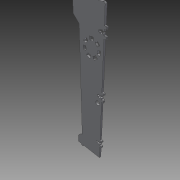
# Autodesk Inventor part: inner_brace_right
Saved by Autodesk Inventor 2014 (Build 180170000, 170)
## iProperties
Created: 2014-03-31
Part Number: inner_brace_right
Material: Plywood, Finish
Document SubType Name: Modeling
Designer: buben
Density: 0.552 g/cm^3
Appearance: Plywood - New
Author: buben
Autodesk Inventor part; units mm, degrees
ref_plane "YZ Plane" through (0, 0, 0) normal (1, 0, 0) x (0, 1, 0)
ref_plane "XZ Plane" through (0, 0, 0) normal (0, 1, 0) x (-1, 0, 0)
ref_plane "XY Plane" through (0, 0, 0) normal (0, 0, 1) x (1, 0, 0)
sketch "Sketch1" plane through (0, 0, 0) normal (0, 1, 0) x (-1, 0, 0)
  line L0 (0, 0) -> (-100, 0)
  line L1 (-100, 0) -> (-100, -489)
  line L2 (-100, -489) -> (0, -489)
  line L3 (0, -489) -> (0, 0)
  dimension "d0" = 489
  dimension "d1" = 100
  constraints: 8 end point, 2 parallel, 1 horizontal, 1 perpendicular
  measures "d0" distance of L2.end L0.start
  measures "d1" distance of L0.start L0.end
extrude "Extrusion1" add sketch "Sketch1" along normal blind 6.5
sketch "Sketch2" plane through (0, 6.5, 0) normal (0, 1, 0) x (1, 0, 0)
  line L0 (0, 489) -> (0, 0) projected
  line L1 (0, 459) -> (20, 439)
  line L2 (20, 439) -> (20, 65)
  line L3 (20, 65) -> (0, 45)
  line L4 (0, 459) -> (0, 45)
  dimension "d4" = 45
  dimension "d5" = 20
  dimension "d6" = 30
  dimension "d7" = 45
  constraints: 8 end point, 2 parallel, 2 point on line, 1 perpendicular
  measures "d4" angle of L0 L1
  measures "d5" distance between parallel lines of L0 L2
  measures "d6" distance of L0.start L1.start
  measures "d7" distance of L0.end L3.end
extrude "Extrusion2" cut sketch "Sketch2" against normal through all
sketch "Sketch3" plane through (0, 6.5, 0) normal (0, 1, 0) x (1, 0, 0)
  line L0 (0, 0) -> (100, 0) projected
  line L1 (100, 0) -> (100, 489) projected
  line L2 (100, 489) -> (0, 489) projected
  line L3 (100, 425.75) -> (100, 421.25)
  line L4 (83.7, 421.25) -> (83.7, 425.75)
  line L5 (87.7, 428.25) -> (95, 428.25)
  line L6 (95, 418.75) -> (87.7, 418.75)
  line L7 (83.7, 425.75) -> (87.7, 425.75)
  line L8 (95, 425.75) -> (100, 425.75)
  line L9 (87.7, 418.75) -> (87.7, 421.25)
  line L10 (87.7, 425.75) -> (87.7, 428.25)
  line L11 (100, 421.25) -> (95, 421.25)
  line L12 (87.7, 421.25) -> (83.7, 421.25)
  line L13 (95, 428.25) -> (95, 425.75)
  line L14 (95, 421.25) -> (95, 418.75)
  line L15 (100, 246.75) -> (100, 242.25)
  line L16 (83.7, 242.25) -> (83.7, 246.75)
  line L17 (87.7, 249.25) -> (95, 249.25)
  line L18 (95, 239.75) -> (87.7, 239.75)
  line L19 (83.7, 246.75) -> (87.7, 246.75)
  line L20 (95, 246.75) -> (100, 246.75)
  line L21 (87.7, 239.75) -> (87.7, 242.25)
  line L22 (87.7, 246.75) -> (87.7, 249.25)
  line L23 (100, 242.25) -> (95, 242.25)
  line L24 (87.7, 242.25) -> (83.7, 242.25)
  line L25 (95, 249.25) -> (95, 246.75)
  line L26 (95, 242.25) -> (95, 239.75)
  line L27 (100, 67.75) -> (100, 63.25)
  line L28 (83.7, 63.25) -> (83.7, 67.75)
  line L29 (87.7, 70.25) -> (95, 70.25)
  line L30 (95, 60.75) -> (87.7, 60.75)
  line L31 (83.7, 67.75) -> (87.7, 67.75)
  line L32 (95, 67.75) -> (100, 67.75)
  line L33 (87.7, 60.75) -> (87.7, 63.25)
  line L34 (87.7, 67.75) -> (87.7, 70.25)
  line L35 (100, 63.25) -> (95, 63.25)
  line L36 (87.7, 63.25) -> (83.7, 63.25)
  line L37 (95, 70.25) -> (95, 67.75)
  line L38 (95, 63.25) -> (95, 60.75)
  line L39 (91.35, 418.75) -> (91.35, 249.25) construction
  line L40 (91.35, 239.75) -> (91.35, 70.25) construction
  point P0 (83.7, 423.5)
  point P1 (83.7, 244.5)
  point P2 (83.7, 65.5)
  dimension "d10" = 4.5
  dimension "d11" = 5
  dimension "d12" = 4
  dimension "d13" = 7.3
  dimension "d14" = 2.5
  dimension "d15" = 4.5
  dimension "d16" = 5
  dimension "d17" = 4
  dimension "d18" = 7.3
  dimension "d19" = 2.5
  dimension "d20" = 4.5
  dimension "d21" = 5
  dimension "d22" = 4
  dimension "d23" = 7.3
  dimension "d24" = 2.5
  dimension "d25" = 65.5
  dimension "d26" = 65.5
  constraints: 76 end point, 30 parallel, 19 collinear, 12 perpendicular, 9 horizontal, 7 midpoint
  measures "d10" distance of L4.start L4.end
  measures "d11" distance of L3.end L11.end
  measures "d12" distance of L9.end L4.start
  measures "d13" distance of L6.start L6.end
  measures "d14" distance of L6.end L9.end
  measures "d15" distance of L24.end L16.end
  measures "d16" distance of L15.end L23.end
  measures "d17" distance of L21.end L24.end
  measures "d18" distance of L26.end L21.start
  measures "d19" distance of L21.start L21.end
  measures "d20" distance of L36.end L28.end
  measures "d21" distance of L27.end L35.end
  measures "d22" distance of L33.end L36.end
  measures "d23" distance of L38.end L33.start
  measures "d24" distance of L33.start L33.end
  measures "d25" distance from line of L2 point (83.7, 423.5)
  measures "d26" distance from line of L0 point (83.7, 65.5)
extrude "Extrusion3" cut sketch "Sketch3" against normal through all
sketch "Sketch4" plane through (0, 6.5, 0) normal (0, 1, 0) x (1, 0, 0)
  line L0 (83.7, 242.25) -> (83.7, 246.75) projected
  line L1 (100, 246.75) -> (100, 421.25) projected
  line L2 (83.7, 421.25) -> (83.7, 425.75) projected
  line L3 (100, 425.75) -> (100, 489) projected
  line L4 (100, 0) -> (100, 63.25) projected
  line L5 (83.7, 63.25) -> (83.7, 67.75) projected
  line L6 (100, 67.75) -> (100, 242.25) projected
  line L7 (100, 439) -> (104.5, 439)
  line L8 (106.5, 437) -> (106.5, 433)
  line L9 (104.5, 431) -> (100, 431)
  line L10 (100, 431) -> (100, 439)
  line L11 (100, 416) -> (104.5, 416)
  line L12 (106.5, 414) -> (106.5, 410)
  line L13 (104.5, 408) -> (100, 408)
  line L14 (100, 408) -> (100, 416)
  line L15 (100, 260) -> (104.5, 260)
  line L16 (106.5, 258) -> (106.5, 254)
  line L17 (104.5, 252) -> (100, 252)
  line L18 (100, 252) -> (100, 260)
  line L19 (100, 237) -> (104.5, 237)
  line L20 (106.5, 235) -> (106.5, 231)
  line L21 (104.5, 229) -> (100, 229)
  line L22 (100, 229) -> (100, 237)
  line L23 (100, 81) -> (104.5, 81)
  line L24 (106.5, 79) -> (106.5, 75)
  line L25 (104.5, 73) -> (100, 73)
  line L26 (100, 73) -> (100, 81)
  line L27 (100, 58) -> (104.5, 58)
  line L28 (106.5, 56) -> (106.5, 52)
  line L29 (104.5, 50) -> (100, 50)
  line L30 (100, 50) -> (100, 58)
  arc A0 (106.5, 437) -> (104.5, 439) centre (104.5, 437) ccw
  arc A1 (104.5, 431) -> (106.5, 433) centre (104.5, 433) ccw
  arc A2 (106.5, 414) -> (104.5, 416) centre (104.5, 414) ccw
  arc A3 (104.5, 408) -> (106.5, 410) centre (104.5, 410) ccw
  arc A4 (106.5, 258) -> (104.5, 260) centre (104.5, 258) ccw
  arc A5 (104.5, 252) -> (106.5, 254) centre (104.5, 254) ccw
  arc A6 (106.5, 235) -> (104.5, 237) centre (104.5, 235) ccw
  arc A7 (104.5, 229) -> (106.5, 231) centre (104.5, 231) ccw
  arc A8 (106.5, 79) -> (104.5, 81) centre (104.5, 79) ccw
  arc A9 (104.5, 73) -> (106.5, 75) centre (104.5, 75) ccw
  arc A10 (106.5, 56) -> (104.5, 58) centre (104.5, 56) ccw
  arc A11 (104.5, 50) -> (106.5, 52) centre (104.5, 52) ccw
  point P0 (83.7, 423.5)
  point P1 (83.7, 244.5)
  point P2 (83.7, 65.5)
  dimension "d29" = 2
  dimension "d30" = 6.5
  dimension "d31" = 8
  dimension "d32" = 8
  dimension "d33" = 8
  dimension "d34" = 8
  dimension "d37" = 8
  dimension "d38" = 8
  dimension "d39" = 15
  dimension "d40" = 15
  dimension "d41" = 15
  dimension "d42" = 7.5
  dimension "d43" = 7.5
  dimension "d44" = 7.5
  constraints: 48 end point, 24 point on circle, 24 tangent, 12 centre point, 12 parallel, 11 equal radius, 6 horizontal, 6 perpendicular, 6 point on line, 5 collinear, 3 midpoint
  measures "d29" radius of A0
  measures "d30" distance between parallel lines of L3 L8
  measures "d31" distance between parallel lines of L9 L7
  measures "d32" distance between parallel lines of L13 L11
  measures "d33" distance between parallel lines of L17 L15
  measures "d34" distance between parallel lines of L21 L19
  measures "d37" distance between parallel lines of L25 L23
  measures "d38" distance between parallel lines of L29 L27
  measures "d39" distance between parallel lines of L11 L9
  measures "d40" distance between parallel lines of L19 L17
  measures "d41" distance between parallel lines of L27 L25
  measures "d42" distance from line of point (83.7, 423.5) L9
  measures "d43" distance from line of point (83.7, 244.5) L17
  measures "d44" distance from line of point (83.7, 65.5) L25
extrude "Extrusion4" add sketch "Sketch4" against normal blind 6.5
sketch "Sketch5" plane through (0, 6.5, 0) normal (0, 1, 0) x (1, 0, 0)
  line L0 (100, 489) -> (0, 489) projected
  line L1 (0, 489) -> (0, 459) projected
  line L2 (0, 45) -> (0, 0) projected
  line L3 (0, 0) -> (100, 0) projected
  line L4 (15, 489) -> (23, 489)
  line L5 (23, 489) -> (23, 493.5)
  line L6 (21, 495.5) -> (17, 495.5)
  line L7 (15, 493.5) -> (15, 489)
  line L8 (15, 0) -> (23, 0)
  line L9 (23, 0) -> (23, -4.5)
  line L10 (21, -6.5) -> (17, -6.5)
  line L11 (15, -4.5) -> (15, 0)
  arc A0 (15, -4.5) -> (17, -6.5) centre (17, -4.5) ccw
  arc A1 (21, -6.5) -> (23, -4.5) centre (21, -4.5) ccw
  arc A2 (23, 493.5) -> (21, 495.5) centre (21, 493.5) ccw
  arc A3 (17, 495.5) -> (15, 493.5) centre (17, 493.5) ccw
  dimension "d47" = 2
  dimension "d48" = 8
  dimension "d49" = 6.5
  dimension "d50" = 15
  dimension "d51" = 8
  dimension "d52" = 6.5
  dimension "d53" = 15
  constraints: 16 end point, 8 point on circle, 8 tangent, 4 centre point, 4 parallel, 3 equal radius, 2 horizontal, 2 perpendicular, 2 point on line
  measures "d47" radius of A0
  measures "d48" distance between parallel lines of L5 L7
  measures "d49" distance between parallel lines of L0 L6
  measures "d50" distance between parallel lines of L1 L7
  measures "d51" distance between parallel lines of L9 L11
  measures "d52" distance between parallel lines of L3 L10
  measures "d53" distance between parallel lines of L2 L11
extrude "Extrusion5" add sketch "Sketch5" against normal blind 6.5
sketch "Sketch6" plane through (0, 6.5, 0) normal (0, 1, 0) x (1, 0, 0)
  line L0 (100, 237) -> (100, 242.25) projected
  circle A0 centre (62, 115) radius 30 construction
  arc A1 (44.6795, 125) -> (42, 115) centre (62, 115) ccw
  arc A2 (36.0192, 130) -> (32, 115) centre (62, 115) ccw
  line L1 (42, 115) -> (32, 115)
  line L2 (44.6795, 125) -> (36.0192, 130)
  arc A3 (43.3825, 107.6932) -> (49.5302, 99.3634) centre (62, 115) ccw
  arc A4 (34.0738, 104.0398) -> (43.2953, 91.5451) centre (62, 115) ccw
  line L3 (49.5302, 99.3634) -> (43.2953, 91.5451)
  line L4 (43.3825, 107.6932) -> (34.0738, 104.0398)
  arc A5 (56.1049, 95.8885) -> (66.4504, 95.5014) centre (62, 115) ccw
  arc A6 (53.1573, 86.3328) -> (68.6756, 85.7522) centre (62, 115) ccw
  line L5 (66.4504, 95.5014) -> (68.6756, 85.7522)
  line L6 (56.1049, 95.8885) -> (53.1573, 86.3328)
  arc A7 (73.2664, 98.4752) -> (80.0194, 106.3223) centre (62, 115) ccw
  arc A8 (78.8996, 90.2128) -> (89.0291, 101.9835) centre (62, 115) ccw
  line L7 (80.0194, 106.3223) -> (89.0291, 101.9835)
  line L8 (73.2664, 98.4752) -> (78.8996, 90.2128)
  arc A9 (81.9441, 113.5054) -> (80.0194, 123.6777) centre (62, 115) ccw
  arc A10 (91.9161, 112.7581) -> (89.0291, 128.0165) centre (62, 115) ccw
  line L9 (80.0194, 123.6777) -> (89.0291, 128.0165)
  line L10 (81.9441, 113.5054) -> (91.9161, 112.7581)
  arc A11 (75.6035, 129.661) -> (66.4504, 134.4986) centre (62, 115) ccw
  arc A12 (82.4052, 136.9916) -> (68.6756, 144.2478) centre (62, 115) ccw
  line L11 (66.4504, 134.4986) -> (68.6756, 144.2478)
  line L12 (75.6035, 129.661) -> (82.4052, 136.9916)
  arc A13 (59.0192, 134.7766) -> (49.5302, 130.6366) centre (62, 115) ccw
  arc A14 (57.5287, 144.6649) -> (43.2953, 138.4549) centre (62, 115) ccw
  line L13 (49.5302, 130.6366) -> (43.2953, 138.4549)
  line L14 (59.0192, 134.7766) -> (57.5287, 144.6649)
  line L15 (100, 81) -> (100, 229) projected
  line L16 (23, 0) -> (100, 0) projected
  dimension "d56" = 60
  dimension "d57" = 30
  dimension "d59" = 20
  dimension "d62" = 360
  dimension "d72" = 38
  dimension "d74" = 30
  dimension "d75" = 115
  constraints: 28 end point, 28 point on circle, 16 coincident, 15 centre point, 2 line through centre, 1 perpendicular, 76 other
  measures "d56" diameter of A0
  measures "d57" angle of L1 L2
  measures "d59" radius of A1
  measures "d72" distance from line of L15 A0.centre
  measures "d74" radius of A2
  measures "d75" distance from line of A0.centre L16
extrude "Extrusion6" cut sketch "Sketch6" against normal through all
chamfer "Chamfer1" distance 2 angle 45 14 edges at (36.0192, 3.25, -130) (32, 3.25, -115) (43.2953, 3.25, -138.4549) (57.5287, 3.25, -144.6649) (68.6756, 3.25, -144.2478) (82.4052, 3.25, -136.9916) (89.0291, 3.25, -128.0165) (91.9161, 3.25, -112.7581) (78.8996, 3.25, -90.2128) (89.0291, 3.25, -101.9835) (68.6756, 3.25, -85.7522) (53.1573, 3.25, -86.3328) (43.2953, 3.25, -91.5451) (34.0738, 3.25, -104.0398)
chamfer "Chamfer2" distance 1 angle 45 14 edges at (43.3825, 3.25, -107.6932) (49.5302, 3.25, -99.3634) (56.1049, 3.25, -95.8885) (66.4504, 3.25, -95.5014) (73.2664, 3.25, -98.4752) (80.0194, 3.25, -106.3223) (81.9441, 3.25, -113.5054) (80.0194, 3.25, -123.6777) (42, 3.25, -115) (44.6795, 3.25, -125) (49.5302, 3.25, -130.6366) (59.0192, 3.25, -134.7766) (66.4504, 3.25, -134.4986) (75.6035, 3.25, -129.661)
sketch "Sketch7" plane through (0, 6.5, 0) normal (0, 1, 0) x (1, 0, 0)
  arc A0 (80.8945, 138.3023) -> (70.6096, 143.738) centre (62, 115) ccw projected
  line L0 (100, 260) -> (100, 408) projected
  circle A1 centre (86, 270) radius 7.5
  dimension "d76" = 15
  dimension "d77" = 14
  dimension "d78" = 155
  constraints: 1 centre point
  measures "d76" diameter of A1
  measures "d77" distance from line of L0 A1.centre
  measures "d78" vertical distance of A0.centre A1.centre
extrude "Extrusion7" cut sketch "Sketch7" against normal through all
chamfer "Chamfer3" distance 4 angle 45 1 edges at (100, 3.25, 0)
equation "\"d26\" = d25"
equation "\"d32\" = d31"
equation "\"d33\" = d32"
equation "\"d34\" = d33"
equation "\"d37\" = d34"
equation "\"d38\" = d37"
equation "\"d42\" = 0.5 * d39"
equation "\"d43\" = 0.5 * d40"
equation "\"d44\" = 0.5 * d41"
equation "\"d51\" = d48"
equation "\"d52\" = d49"
equation "\"d53\" = d50"
body "Solid1"
